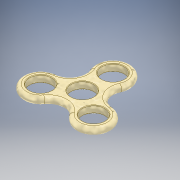
# Autodesk Inventor part: TO4
Saved by Autodesk Inventor 2018 (Build 220112000, 112)
## iProperties
Created: 2020-06-26
Part Number: TO4
Material: Generic
Document SubType Name: Modeling
Designer: Brandon Portillo
Density: 1 g/cm^3
Appearance: Fine - Cream
Author: Brandon Portillo
Autodesk Inventor part; units mm, degrees
ref_plane "YZ Plane" through (0, 0, 0) normal (1, 0, 0) x (0, 1, 0)
ref_plane "XZ Plane" through (0, 0, 0) normal (0, 1, 0) x (-1, 0, 0)
ref_plane "XY Plane" through (0, 0, 0) normal (0, 0, 1) x (1, 0, 0)
sketch "Sketch1" plane through (0, 0, 0) normal (0, 0, 1) x (1, 0, 0)
  circle A0 centre (0, 0) radius 11
  circle A1 centre (0, 30) radius 11
  circle A2 centre (-25.9808, -15) radius 11
  circle A3 centre (25.9808, -15) radius 11
  circle A4 centre (0, 30) radius 17
  circle A5 centre (-25.9808, -15) radius 17
  circle A6 centre (25.9808, -15) radius 17
  arc A7 (-27.6746, 1.9154) -> (-15.4961, 23.0092) centre (-29.1691, 16.8408) ccw
  arc A8 (15.4961, 23.0092) -> (27.6746, 1.9154) centre (29.1691, 16.8408) ccw
  arc A9 (12.1785, -24.9246) -> (-12.1785, -24.9246) centre (0, -33.6815) ccw
  dimension "d0" = 22
  dimension "d1" = 22
  dimension "d2" = 30
  dimension "d5" = 360
  dimension "d7" = 6
  dimension "d8" = 6
  dimension "d9" = 6
  dimension "d10" = 15
  dimension "d11" = 15
  dimension "d12" = 15
  constraints: 12 point on circle, 10 centre point, 6 tangent, 1 coincident, 1 vertical alignment, 7 other
  measures "d0" diameter of A0
  measures "d1" diameter of A1
  measures "d2" distance of A1.centre point (0, 0)
  measures "d7" radial gap between concentric circles of A1 A4
  measures "d8" radial gap between concentric circles of A2 A5
  measures "d9" radial gap between concentric circles of A3 A6
  measures "d10" radius of A7
  measures "d11" radius of A8
  measures "d12" radius of A9
extrude "Extrusion1" add sketch "Sketch1" along normal mid plane 7
full round fillet "Fillet1" first side at (17.2542, -0.5688, 3.5) centre faces at (-15.0522, 21.9116, -1.1667) (8.8565, -21.5753, 1.1667) second side at (17.2542, -0.5688, -3.5)
fillet "Fillet2" radius 0.5 8 edges at (-11, 30, -3.5) (-11, 30, 3.5) (-11, 0, -3.5) (-11, 0, 3.5) (14.9808, -15, -3.5) (14.9808, -15, 3.5) (-36.9808, -15, -3.5) (-36.9808, -15, 3.5)
body "Solid1"
